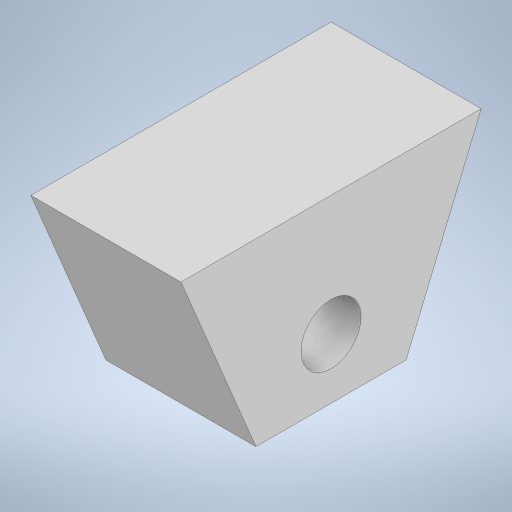
# Autodesk Inventor part: Задание номер 2
Saved by Autodesk Inventor 2023.2 (Build 272271030, 271C)
## iProperties
Created: 2023-09-07
Part Number: Задание номер 2
Material: Типовые
Document SubType Name: Modeling
Designer: User
Density: 1 g/cm^3
Appearance: По умолчанию
Author: User
Autodesk Inventor part; units mm, degrees
ref_plane "YZ Plane" through (0, 0, 0) normal (1, 0, 0) x (0, 1, 0)
ref_plane "XZ Plane" through (0, 0, 0) normal (0, 1, 0) x (-1, 0, 0)
ref_plane "XY Plane" through (0, 0, 0) normal (0, 0, 1) x (1, 0, 0)
sketch "Эскиз1" plane through (0, 0, 0) normal (1, 0, 0) x (0, 1, 0)
  line L0 (28.6824, 20.6548) -> (28.6824, -19.3452)
  line L1 (28.6824, -19.3452) -> (28.6824, 20.6548)
  line L2 (4.6824, 0.6548) -> (4.6824, 10.6548)
  line L3 (4.6824, 0.6548) -> (4.6824, -9.3452)
  line L4 (28.6824, -19.3452) -> (4.6824, -9.3452)
  line L5 (4.6824, 10.6548) -> (28.6824, 20.6548)
  circle A0 centre (12.6824, 0.6548) radius 4
  dimension "d0" = 40
  dimension "d1" = 10
  dimension "d2" = 10
  dimension "d3" = 8
  constraints: 12 end point, 2 vertical, 1 centre point, 1 collinear
  measures "d0" distance of L0.start L0.end
  measures "d1" distance of L2.start L2.end
  measures "d2" distance of L2.start L3.end
  measures "d3" diameter of A0
extrude "Выдавливание1" add sketch "Эскиз1" along normal blind 20
